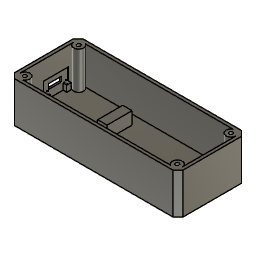
Deej-2024-03-25 v40 (Autodesk Fusion 360 design; units mm, degrees)
Autodesk Fusion 360 part; units mm, degrees
sketch "Sketch1" plane through (0, 0, 0) normal (0, 0, 1) x (1, 0, 0)
  line L0 (0, 0) -> (135, 0)
  line L1 (135, 0) -> (135, 55)
  line L2 (135, 55) -> (0, 55)
  line L3 (0, 55) -> (0, 0)
  dimension "d1" = 135
  dimension "d2" = 55
  constraint horizontal L0
  constraint vertical L1
  constraint horizontal L2
  constraint vertical L3
  constraint coincident L0.start L3.end
  measures "d1" distance of L0.start L0.end
  measures "d2" distance of L0.start L2.end
extrude "Extrude1" add sketch "Sketch1" along normal blind 3.5 makes body 1
chamfer "Chamfer1" distance 4 angle 45 4 edges at (135, 55, 1.75) (135, 0, 1.75) (0, 0, 1.75) (0, 55, 1.75) on bodies 1
chamfer "Chamfer2" distance 2 angle 45 1 faces at (46.3333, 36.6667, 3.5) on bodies 1
sketch "Sketch2" plane through (0, 0, 3.5) normal (0, 0, 1) x (-1, 0, 0)
  line L0 (-4.8284, -2) -> (-130.1716, -2)
  line L1 (-130.1716, -2) -> (-133, -4.8284)
  line L2 (-133, -4.8284) -> (-133, -50.1716)
  line L3 (-133, -50.1716) -> (-130.1716, -53)
  line L4 (-130.1716, -53) -> (-4.8284, -53)
  line L5 (-4.8284, -53) -> (-2, -50.1716)
  line L6 (-2, -50.1716) -> (-2, -4.8284)
  line L7 (-2, -4.8284) -> (-4.8284, -2)
  line L8 (-2, -27.5) -> (-133, -27.5)
  constraint midpoint L6 L8.start
  constraint midpoint L2 L8.end
sketch "Sketch3" plane through (0, 0, 3.5) normal (0, 0, 1) x (1, 0, 0)
  line L0 (2, 27.5) -> (133, 27.5)
  circle A0 centre (22.5, 40.25) radius 3.6
  circle A1 centre (52.5, 40.25) radius 3.6
  circle A2 centre (82.5, 40.25) radius 3.6
  circle A3 centre (112.5, 40.25) radius 3.6
  line L1 (130.1716, 2) -> (4.8284, 2)
  circle A4 centre (112.5, 14.75) radius 7.375
  circle A5 centre (52.5, 14.75) radius 7.375
  circle A6 centre (22.5, 14.75) radius 7.375
  circle A7 centre (82.5, 14.75) radius 7.375
  line L2 (4.8284, 53) -> (130.1716, 53)
  line L3 (4.8284, 2) -> (130.1716, 2)
  line L4 (135, 0) -> (135, 55)
  line L5 (0, 55) -> (0, 0)
  line L6 (130.1716, 53) -> (4.8284, 53)
  point P0 (2, 27.5)
  point P1 (130.1716, 2)
  point P2 (4.8284, 2)
  dimension "d18" = 7.2
  dimension "d19" = 30
  dimension "d20" = 7.2
  dimension "d21" = 30
  dimension "d22" = 7.2
  dimension "d23" = 30
  dimension "d24" = 7.2
  dimension "d116" = 14.75
  dimension "d117" = 30
  dimension "d118" = 14.75
  dimension "d119" = 30
  dimension "d120" = 14.75
  dimension "d121" = 30
  dimension "d122" = 14.75
  dimension "d219" = 25.5
  measures "d18" diameter of A0
  measures "d19" distance of A0.centre A1.centre
  measures "d20" diameter of A1
  measures "d21" distance of A1.centre A2.centre
  measures "d22" diameter of A2
  measures "d23" distance of A2.centre A3.centre
  measures "d24" diameter of A3
  measures "d116" diameter of A6
  measures "d117" distance of A5.centre A6.centre
  measures "d118" diameter of A5
  measures "d119" distance of A5.centre A7.centre
  measures "d120" diameter of A7
  measures "d121" distance of A7.centre A4.centre
  measures "d122" diameter of A4
  measures "d219" distance of A0.centre A6.centre
extrude "Extrude26" cut sketch "Sketch3" against normal blind 3.5 bodies 1
sketch "Sketch4" plane through (0, 0, 0) normal (0, 0, -1) x (1, 0, 0)
  line L0 (0, -51) -> (4, -55)
  line L1 (4, -55) -> (131, -55)
  line L2 (131, -55) -> (135, -51)
  line L3 (135, -51) -> (135, -4)
  line L4 (135, -4) -> (131, 0)
  line L5 (131, 0) -> (4, 0)
  line L6 (4, 0) -> (0, -4)
  line L7 (0, -4) -> (0, -51)
  circle A0 centre (52.5, -14.75) radius 7.375
  circle A1 centre (22.5, -40.25) radius 3.6
  circle A2 centre (52.5, -40.25) radius 3.6
  circle A3 centre (82.5, -14.75) radius 7.375
  circle A4 centre (112.5, -14.75) radius 7.375
  circle A5 centre (112.5, -40.25) radius 3.6
  circle A6 centre (82.5, -40.25) radius 3.6
  circle A7 centre (22.5, -14.75) radius 7.375
  circle A8 centre (112.5, -48.25) radius 1.5
  circle A9 centre (82.5, -48.25) radius 1.5
  circle A10 centre (52.5, -48.25) radius 1.5
  circle A11 centre (22.5, -48.25) radius 1.5
  circle A12 centre (82.5, -32.25) radius 1.5
  circle A13 centre (112.5, -32.25) radius 1.5
  circle A14 centre (52.5, -32.25) radius 1.5
  circle A15 centre (22.5, -32.25) radius 1.5
  point P0 (22.5, -40.25)
  point P1 (52.5, -40.25)
  point P2 (52.5, -40.25)
  dimension "d191" = 3
  dimension "d193" = 3
  dimension "d194" = 3
  dimension "d195" = 3
  dimension "d196" = 3
  dimension "d197" = 3
  dimension "d198" = 3
  dimension "d199" = 3
  measures "d191" diameter of A8
  measures "d193" diameter of A9
  measures "d194" diameter of A10
  measures "d195" diameter of A11
  measures "d196" diameter of A12
  measures "d197" diameter of A13
  measures "d198" diameter of A14
  measures "d199" diameter of A15
extrude "Extrude29" cut sketch "Sketch4" against normal blind 1.75 contours A8 | A9 | A10 | A11 | A12 | A13 | A14 | A15 bodies 1
sketch "Sketch5" plane through (0, 0, 3.5) normal (0, 0, 1) x (-1, 0, 0)
  line L0 (-4.8284, -2) -> (-130.1716, -2)
  line L1 (-130.1716, -2) -> (-133, -4.8284)
  line L2 (-133, -4.8284) -> (-133, -50.1716)
  line L3 (-133, -50.1716) -> (-130.1716, -53)
  line L4 (-130.1716, -53) -> (-4.8284, -53)
  line L5 (-4.8284, -53) -> (-2, -50.1716)
  line L6 (-2, -50.1716) -> (-2, -4.8284)
  line L7 (-2, -4.8284) -> (-4.8284, -2)
  line L8 (-6, -48.5147) -> (-6, -6.4853)
  line L9 (-6, -6.4853) -> (-6.4853, -6)
  line L10 (-6.4853, -6) -> (-128.5147, -6)
  line L11 (-128.5147, -6) -> (-129, -6.4853)
  line L12 (-129, -6.4853) -> (-129, -48.5147)
  line L13 (-129, -48.5147) -> (-128.5147, -49)
  line L14 (-128.5147, -49) -> (-6.4853, -49)
  line L15 (-6.4853, -49) -> (-6, -48.5147)
  circle A0 centre (-52.5, -14.75) radius 7.375
  circle A1 centre (-22.5, -40.25) radius 3.6
  circle A2 centre (-52.5, -40.25) radius 3.6
  circle A3 centre (-82.5, -14.75) radius 7.375
  circle A4 centre (-112.5, -14.75) radius 7.375
  circle A5 centre (-112.5, -40.25) radius 3.6
  circle A6 centre (-82.5, -40.25) radius 3.6
  circle A7 centre (-22.5, -14.75) radius 7.375
  dimension "d37" = -4
hole "Hole1" at (6.4853, 6, 3.5) direction (0, 0, -1) diameter 3 depth 20.35 tip angle 118 countersink diameter 4.5 countersink angle 90 bodies 1
hole "Hole2" at (128.5147, 6, 3.5) direction (0, 0, -1) diameter 3 depth 20.35 tip angle 118 countersink diameter 4.5 countersink angle 90 bodies 1
hole "Hole3" at (128.5147, 49, 3.5) direction (0, 0, -1) diameter 3 depth 20.35 tip angle 118 countersink diameter 4.5 countersink angle 90 bodies 1
hole "Hole4" at (6.4853, 49, 3.5) direction (0, 0, -1) diameter 3 depth 20.35 tip angle 118 countersink diameter 4.5 countersink angle 90 bodies 1
extrude "Extrude5" add 1 faces at (100.6911, 27.9466, 0) along direction (0, 0, -1) blind 32.5 separate body on bodies 1 makes body 2
sketch "Sketch6" plane through (0, 0, -32.5) normal (0, 0, -1) x (1, 0, 0)
  line L0 (0, -51) -> (4, -55)
  line L1 (4, -55) -> (131, -55)
  line L2 (131, -55) -> (135, -51)
  line L3 (135, -51) -> (135, -4)
  line L4 (135, -4) -> (131, 0)
  line L5 (131, 0) -> (4, 0)
  line L6 (4, 0) -> (0, -4)
  line L7 (0, -4) -> (0, -51)
  circle A0 centre (6.4853, -49) radius 1.5
  circle A1 centre (128.5147, -49) radius 1.5
  circle A2 centre (128.5147, -6) radius 1.5
  circle A3 centre (6.4853, -6) radius 1.5
  arc A4 (2.5, -5.6572) -> (8.4218, -2.5) centre (6.4853, -6) ccw
  arc A5 (8.4218, -52.5) -> (2.5, -49.3428) centre (6.4853, -49) ccw
  line L8 (2.5, -5.6572) -> (2.5, -49.3428)
  line L9 (2.5, -52.5) -> (2.5, -52.5179)
  arc A6 (132.5, -49.3428) -> (126.5782, -52.5) centre (128.5147, -49) ccw
  line L10 (8.4218, -52.5) -> (126.5782, -52.5)
  line L11 (132.5, -49.3428) -> (132.5, -5.6572)
  line L12 (132.5, -2.5) -> (132.5, -2.4416)
  arc A7 (126.5782, -2.5) -> (132.5, -5.6572) centre (128.5147, -6) ccw
  line L13 (126.5782, -2.5) -> (8.4218, -2.5)
  dimension "d165" = 130
  dimension "d166" = 2.5
  dimension "d207" = 2.5
  dimension "d211" = 6.4853
  dimension "d212" = 2.5
  constraint parallel L7 L8
  constraint parallel L3 L11
  constraint concentric A3 A4
  constraint concentric A0 A5
  constraint concentric A1 A6
  constraint concentric A2 A7
  constraint collinear L8 L9
  constraint collinear L11 L12
  measures "d165" distance of L8 L11
  measures "d166" distance of L7 L8
  measures "d207" distance of L3 L11
  measures "d211" distance of L3 A2.centre
  measures "d212" distance of L7 L8
extrude "Extrude6" cut sketch "Sketch6" against normal blind 110 contours A4 A5 L8 A6 L10 L11 A7 L13 bodies 2
extrude "Extrude7" add sketch "Sketch6" against normal blind 2.5 contours A4 A5 L8 A6 L10 L11 A7 L13 bodies 2
extrude "Extrude28" add sketch "Sketch6" against normal blind 2.5 contours A0 | A1 | A2 | A3 bodies 2
sketch "Sketch7" plane through (2.5, 0, 0) normal (1, 0, 0) x (0, 1, 0)
  line L0 (25, -30) -> (45, -30)
  line L1 (45, -30) -> (45, -15)
  line L2 (45, -15) -> (25, -15)
  line L3 (25, -15) -> (25, -30)
  line L4 (48.6572, -30) -> (48.6572, 0)
  line L5 (6.3428, 0) -> (6.3428, -30)
  line L6 (6.3428, -30) -> (48.6572, -30)
  dimension "d81" = 20
  dimension "d82" = 15
  constraint vertical L1
  constraint horizontal L2
  constraint vertical L3
  measures "d81" distance of L0.start L0.end
  measures "d82" distance of L0.start L2.end
extrude "Extrude11" cut sketch "Sketch7" against normal blind 1 bodies 2
sketch "Sketch8" plane through (1.5, 0, 0) normal (1, 0, 0) x (0, 1, 0)
  line L0 (30, -19.7) -> (40, -19.7)
  line L1 (40, -19.7) -> (40, -23.7)
  line L2 (40, -23.7) -> (30, -23.7)
  line L3 (30, -23.7) -> (30, -19.7)
  line L4 (30, -19.7) -> (35, -19.7)
  point P0 (25, -15)
  dimension "d90" = 4
  dimension "d164" = 10
  dimension "d275" = 5
  constraint perpendicular L3 L4
  measures "d90" distance of L0.start L2.end
  measures "d164" distance of L0.start L0.end
  measures "d275" distance of L0.start L4.end
extrude "Extrude12" cut sketch "Sketch8" against normal blind 1.5 bodies 2
sketch "Sketch9" plane through (0, 0, -30) normal (0, 0, 1) x (-1, 0, 0)
  line L0 (-126.5782, -52.5) -> (-8.4218, -52.5)
  line L1 (-2.5, -48.6572) -> (-2.5, -45)
  line L2 (-8.4218, -2.5) -> (-126.5782, -2.5)
  line L3 (-132.5, -6.3428) -> (-132.5, -48.6572)
  arc A0 (-126.5782, -52.5) -> (-132.5, -48.6572) centre (-128.5147, -49) ccw
  arc A1 (-2.5, -48.6572) -> (-8.4218, -52.5) centre (-6.4853, -49) ccw
  arc A2 (-8.4218, -2.5) -> (-2.5, -6.3428) centre (-6.4853, -6) ccw
  arc A3 (-132.5, -6.3428) -> (-126.5782, -2.5) centre (-128.5147, -6) ccw
  circle A4 centre (-43.89, -42.5) radius 0.65
  circle A5 centre (-3.25, -42.5) radius 0.65
  circle A6 centre (-3.25, -27.26) radius 0.65
  circle A7 centre (-43.89, -27.26) radius 0.65
  line L4 (-42.89, -41.5) -> (-45.89, -41.5)
  line L5 (-45.89, -41.5) -> (-45.89, -44.9)
  line L6 (-45.89, -44.9) -> (-42.89, -44.9)
  line L7 (-42.89, -44.9) -> (-42.89, -41.5)
  line L8 (-45.89, -24.86) -> (-42.89, -24.86)
  line L9 (-42.89, -24.86) -> (-42.89, -28.26)
  line L10 (-45.89, -28.26) -> (-45.89, -24.86)
  line L11 (-42.89, -28.26) -> (-45.89, -28.26)
  line L12 (-1.5, -45) -> (-4.5, -45)
  line L13 (-4.5, -45) -> (-4.5, -41.5)
  line L14 (-4.5, -41.5) -> (-1.5, -41.5)
  line L15 (-1.5, -41.5) -> (-1.5, -45)
  line L16 (-1.5, -25) -> (-4.5, -25)
  line L17 (-4.5, -25) -> (-4.5, -28.3)
  line L18 (-4.5, -28.3) -> (-1.5, -28.3)
  line L19 (-1.5, -28.3) -> (-1.5, -25)
  line L20 (-1.5, -45) -> (-1.5, -25)
  line L21 (-1.5, -25) -> (-2.5, -25)
  line L22 (-2.5, -25) -> (-2.5, -6.3428)
  dimension "d244" = 1.3
  dimension "d245" = 1.3
  dimension "d246" = 1.3
  dimension "d247" = 1.3
  constraint horizontal L4
  constraint vertical L5
  constraint horizontal L6
  constraint vertical L7
  constraint horizontal L12
  constraint vertical L13
  constraint horizontal L14
  constraint vertical L15
  constraint horizontal L16
  constraint vertical L17
  constraint horizontal L18
  constraint vertical L19
  measures "d244" diameter of A4
  measures "d245" diameter of A5
  measures "d246" diameter of A7
  measures "d247" diameter of A6
extrude "Extrude38" add sketch "Sketch9" along normal blind 7.5 contours A4 | A5 | A6 | A7 bodies 2
extrude "Extrude39" add sketch "Sketch9" along normal blind 5 contours L12 L13 L14 L15 L20 | L16 L17 L18 L19 L20 L21 | L4 L5 L6 L7 | L8 L9 L10 L11 bodies 2
sketch "Sketch17" plane through (0, 0, -30) normal (0, 0, 1) x (-1, 0, 0)
  line L0 (-42.89, -44.9) -> (-45.89, -44.9)
  line L1 (-45.89, -44.9) -> (-45.89, -41.5)
  line L2 (-45.89, -41.5) -> (-42.89, -41.5)
  line L3 (-42.89, -41.5) -> (-42.89, -44.9)
  line L4 (-1.5, -28.3) -> (-4.5, -28.3)
  line L5 (-4.5, -28.3) -> (-4.5, -25)
  line L6 (-4.5, -25) -> (-2.5, -25)
  line L7 (-2.5, -25) -> (-2.5, -6.3428)
  arc A0 (-8.4218, -2.5) -> (-2.5, -6.3428) centre (-6.4853, -6) ccw
  line L8 (-8.4218, -2.5) -> (-126.5782, -2.5)
  arc A1 (-132.5, -6.3428) -> (-126.5782, -2.5) centre (-128.5147, -6) ccw
  line L9 (-132.5, -6.3428) -> (-132.5, -48.6572)
  arc A2 (-126.5782, -52.5) -> (-132.5, -48.6572) centre (-128.5147, -49) ccw
  line L10 (-126.5782, -52.5) -> (-8.4218, -52.5)
  arc A3 (-2.5, -48.6572) -> (-8.4218, -52.5) centre (-6.4853, -49) ccw
  line L11 (-2.5, -48.6572) -> (-2.5, -45)
  line L12 (-2.5, -45) -> (-4.5, -45)
  line L13 (-4.5, -45) -> (-4.5, -41.5)
  line L14 (-4.5, -41.5) -> (-1.5, -41.5)
  line L15 (-1.5, -41.5) -> (-1.5, -28.3)
  line L16 (-42.89, -28.26) -> (-45.89, -28.26)
  line L17 (-45.89, -28.26) -> (-45.89, -24.86)
  line L18 (-45.89, -24.86) -> (-42.89, -24.86)
  line L19 (-42.89, -24.86) -> (-42.89, -28.26)
  line L20 (-45.89, -24.86) -> (-53.39, -24.86)
  line L21 (-53.39, -24.86) -> (-53.39, -44.9)
  line L22 (-53.39, -44.9) -> (-45.89, -44.9)
  line L23 (-45.89, -44.9) -> (-45.89, -24.86)
  dimension "d276" = 7.5
  constraint horizontal L20
  constraint vertical L21
  constraint horizontal L22
  constraint vertical L23
  constraint coincident L17.end L18.start
  measures "d276" distance of L17.end L20.end
extrude "Extrude40" add sketch "Sketch17" along normal blind 10 contours L1 L17 L20 L21 L22 L23 bodies 2
hidden bodies 1
named bodies: "Tapa", "Caja"
